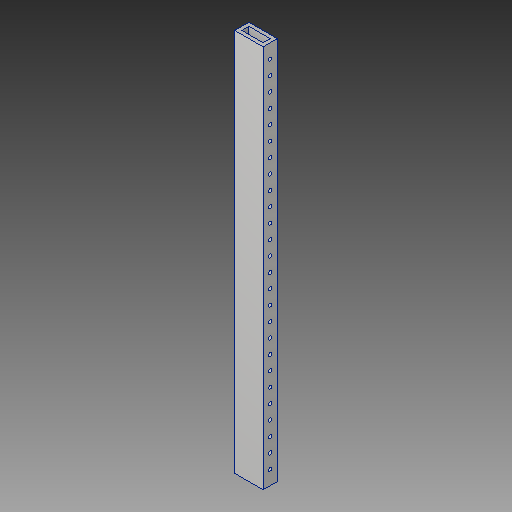
# Autodesk Inventor part: 2AM-17-02-Back Frame
Saved by Autodesk Inventor 2017 (Build 210142000, 142)
## iProperties
Created: 2017-12-28
Part Number: 2AM-17-02-Back Frame
Material: Aluminum 6061
Document SubType Name: Modeling
Designer: anikasoojin
Density: 2.7 g/cm^3
Appearance: Aluminum - Flat
Mass: 1465.04 g
Surface Area: 1791 cm^2
Volume: 542.606 cm^3
Author: anikasoojin
Autodesk Inventor part; units mm, degrees
ref_plane "YZ Plane" through (0, 0, 0) normal (1, 0, 0) x (0, 1, 0)
ref_plane "XZ Plane" through (0, 0, 0) normal (0, 1, 0) x (-1, 0, 0)
ref_plane "XY Plane" through (0, 0, 0) normal (0, 0, 1) x (1, 0, 0)
sketch "Sketch1" plane through (0, 0, 0) normal (0, 0, 1) x (1, 0, 0)
  line L0 (-22.0527, 33.1775) -> (28.7473, 33.1775)
  line L1 (28.7473, 33.1775) -> (28.7473, -652.6225)
  line L2 (28.7473, -652.6225) -> (-22.0527, -652.6225)
  line L3 (-22.0527, -652.6225) -> (-22.0527, 33.1775)
  point P0 (0, 0)
  dimension "d0" = 50.8
  dimension "d1" = 685.8
  constraints: 8 end point, 2 parallel, 1 horizontal, 1 perpendicular
  measures "d0" distance of L0.start L0.end
  measures "d1" distance of L2.end L0.start
extrude "Extrusion1" add sketch "Sketch1" along normal blind 25.4
sketch "Sketch2" plane through (-22.0527, 33.1775, 0) normal (0, 1, 0) x (1, 0, 0)
  line L0 (0, 0) -> (0, -25.4) projected
  line L1 (0, 0) -> (50.8, 0) projected
  line L2 (50.8, 0) -> (50.8, -25.4) projected
  line L3 (50.8, -25.4) -> (0, -25.4) projected
  line L4 (6.35, -19.05) -> (6.35, -6.35)
  line L5 (6.35, -6.35) -> (44.45, -6.35)
  line L6 (44.45, -6.35) -> (44.45, -19.05)
  line L7 (44.45, -19.05) -> (6.35, -19.05)
  point P0 (22.0527, 0)
  dimension "d4" = 6.35
  constraints: 8 end point, 3 other
  measures "d4" distance between parallel lines of L0 L4
extrude "Extrusion2" cut sketch "Sketch2" against normal through all contours L4 L5 L6 L7
sketch "Sketch3" plane through (-22.0527, -652.6225, 0) normal (-1, 0, 0) x (0, 0, 1)
  line L0 (0, 685.8) -> (25.4, 685.8) projected
  line L1 (12.7, 685.8) -> (12.7, 0) construction
  line L2 (6.35, 0) -> (19.05, 0) projected
  circle A0 centre (12.7, 660.4) radius 3.175
  point P0 (0, 652.6225)
  dimension "d7" = 6.35
  dimension "d8" = 25.4
  constraints: 2 end point, 2 midpoint, 1 centre point, 1 point on line
  measures "d7" diameter of A0
  measures "d8" distance of L1.start A0.centre
extrude "Extrusion3" cut sketch "Sketch3" against normal through all
pattern_linear "Rectangular Pattern1" count 26 spacing 25.4 along (0, -1, 0) of "Extrusion3"
body "Solid1"
